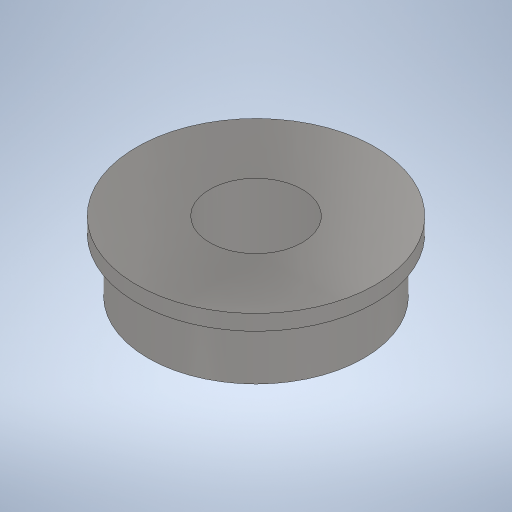
# Autodesk Inventor part: Flange Bearing - 3-8x 7-8x 9-32
Saved by Autodesk Inventor 2023.4 (Build 274418000, 418)
## iProperties
Created: 2024-09-12
Part Number: Flange Bearing - 3-8x 7-8x 9-32
Material: Steel, Alloy
Document SubType Name: Modeling
Designer: Nathan Cai
Density: 7.73 g/cm^3
Appearance: Semi-Polished
Author: Nathan Cai
Autodesk Inventor part; units mm, degrees
ref_plane "YZ Plane" through (0, 0, 0) normal (1, 0, 0) x (0, 1, 0)
ref_plane "XZ Plane" through (0, 0, 0) normal (0, 1, 0) x (-1, 0, 0)
ref_plane "XY Plane" through (0, 0, 0) normal (0, 0, 1) x (1, 0, 0)
sketch "Sketch1" plane through (0, 0, 0) normal (0, 0, 1) x (1, 0, 0)
  line L0 (0, 0) -> (4.7625, 0)
  line L1 (4.7625, 0) -> (4.7625, 7.1437)
  line L2 (4.7625, 7.1437) -> (0, 7.1437)
  line L3 (0, 7.1437) -> (0, 0)
  line L4 (0, 0) -> (11.1125, 0)
  line L5 (11.1125, 0) -> (11.1125, 7.1437)
  line L6 (11.1125, 7.1437) -> (0, 7.1437)
  line L7 (0, 7.1437) -> (0, 0)
  line L8 (11.1125, 7.1437) -> (12.3031, 7.1437)
  line L9 (12.3031, 7.1437) -> (12.3031, 5.5563)
  line L10 (12.3031, 5.5563) -> (11.1125, 5.5563)
  line L11 (11.1125, 5.5563) -> (11.1125, 7.1437)
  dimension "d0" = 4.7625
  dimension "d1" = 7.1437
  dimension "d2" = 11.1125
  dimension "d3" = 7.1437
  dimension "d4" = 12.3031
  dimension "d5" = 1.5875
  constraints: 24 end point, 6 parallel, 3 horizontal, 3 perpendicular
  measures "d0" distance of L2.end L1.end
  measures "d1" distance of L1.end L0.end
  measures "d2" distance of L6.end L5.end
  measures "d3" distance of L5.end L4.end
  measures "d4" distance between parallel lines of L3 L9
  measures "d5" distance between parallel lines of L8 L10
revolve "Revolution1" add sketch "Sketch1" angle 360 about axis through (0, 7.1437, 0) along (0, -1, 0) contours L1 L6 L5 L4 | L8 L9 L10 L5
body "Solid1"
